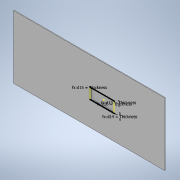
# Autodesk Inventor part: DecupajAgatare
Saved by Autodesk Inventor 2022 (Build 260153000, 153)
## iProperties
Created: 2022-04-14
Part Number: DecupajAgatare
Material: Generic
Document SubType Name: Sheet Metal
Designer: Janina
Density: 1 g/cm^3
Sheet Metal Rule: Default_mm
Appearance: Default
Author: Janina
Autodesk Inventor part; units mm, degrees
ref_plane "YZ Plane" through (0, 0, 0) normal (1, 0, 0) x (0, 1, 0)
ref_plane "XZ Plane" through (0, 0, 0) normal (0, 1, 0) x (-1, 0, 0)
ref_plane "XY Plane" through (0, 0, 0) normal (0, 0, 1) x (1, 0, 0)
sketch "Sketch1" plane through (0, 0, 0) normal (0, 0, 1) x (1, 0, 0)
  line L0 (-71.5423, 25.4266) -> (48.4577, 25.4266)
  line L1 (48.4577, 25.4266) -> (48.4577, -24.5734)
  line L2 (48.4577, -24.5734) -> (-71.5423, -24.5734)
  line L3 (-71.5423, -24.5734) -> (-71.5423, 25.4266)
  point P0 (0, 0)
  dimension "d0" = 50
  dimension "d1" = 120
  measures "d0" distance of L0.end L1.end
  measures "d1" distance of L0.start L0.end
extrude "Plate1" add sketch "Sketch1" along normal blind 0.5
sketch "Sketch2" plane through (0, 0, 0.5) normal (0, 0, 1) x (1, 0, 0)
  line L0 (-11.3208, 3.0189) -> (8.6792, 3.0189)
  line L1 (8.6792, 3.0189) -> (8.6792, -4.9811)
  line L2 (8.6792, -4.9811) -> (-11.3208, -4.9811)
  line L3 (-11.3208, -4.9811) -> (-11.3208, 3.0189)
  point P0 (0, 0)
  point P1 (-1.3208, -0.9811)
  dimension "LG_G" = 20
  dimension "LT_G" = 8
  dimension "d5" = 4
  dimension "d6" = 10
  constraints: 8 end point, 2 parallel, 1 horizontal, 1 perpendicular
  measures "LG_G" distance of L0.start L0.end
  measures "LT_G" distance of L0.end L1.end
  measures "d5" distance from line of L2 point (-1.321, -0.981)
  measures "d6" distance from line of L3 point (-1.321, -0.981)
extrude "Extrusion1" add sketch "Sketch2" against normal blind 1.5
sketch "Sketch3" plane through (0, 0, 0.5) normal (0, 0, 1) x (1, 0, 0)
  line L0 (-11.3208, 3.0189) -> (8.6792, 3.0189) projected
  line L1 (8.6792, 3.0189) -> (8.6792, -4.9811) projected
  line L2 (8.6792, -4.9811) -> (-11.3208, -4.9811) projected
  line L3 (-11.3208, -4.9811) -> (-11.3208, 3.0189) projected
  line L4 (-10.8208, 3.0189) -> (8.1792, 3.0189)
  line L5 (8.1792, 3.0189) -> (8.1792, -4.9811)
  line L6 (8.1792, -4.9811) -> (-10.8208, -4.9811)
  line L7 (-10.8208, -4.9811) -> (-10.8208, 3.0189)
  point P0 (0, 0)
  dimension "d9" = 0.5
  dimension "d10" = 0.5
  constraints: 8 end point, 2 collinear, 2 parallel, 1 horizontal, 1 perpendicular
  measures "d9" distance between parallel lines of L1 L5
  measures "d10" distance between parallel lines of L3 L7
extrude "Extrusion2" cut sketch "Sketch3" against normal blind 1 contours L0 L5 L2 L7
sketch "Sketch4" plane through (0, 0, 0.5) normal (0, 0, 1) x (1, 0, 0)
  line L0 (-10.8208, -4.9811) -> (-10.8208, 3.0189) projected
  line L1 (-10.8208, 3.0189) -> (8.1792, 3.0189) projected
  line L2 (8.1792, 3.0189) -> (8.1792, -4.9811) projected
  line L3 (8.1792, -4.9811) -> (-10.8208, -4.9811) projected
  line L4 (-11.3208, 3.5189) -> (8.6792, 3.5189)
  line L5 (8.6792, 3.5189) -> (8.6792, 3.0189)
  line L6 (8.6792, 3.0189) -> (-11.3208, 3.0189)
  line L7 (-11.3208, 3.0189) -> (-11.3208, 3.5189)
  line L8 (-11.3208, -4.9811) -> (8.6792, -4.9811)
  line L9 (8.6792, -4.9811) -> (8.6792, -5.4811)
  line L10 (8.6792, -5.4811) -> (-11.3208, -5.4811)
  line L11 (-11.3208, -5.4811) -> (-11.3208, -4.9811)
  point P0 (0, 0)
  dimension "d13" = 0.5
  dimension "d14" = 0.5
  dimension "d15" = 0.5
  dimension "d16" = 0.5
  constraints: 16 end point, 4 parallel, 2 collinear, 2 horizontal, 2 perpendicular, 2 point on line
  measures "d13" distance of L4.end L5.end
  measures "d14" distance of L8.end L9.end
  measures "d15" distance between parallel lines of L7 L0
  measures "d16" distance between parallel lines of L2 L5
equation "\"d5\" = 0.5 * LT_G"
equation "\"d6\" = 0.5 * LG_G"
equation "\"d7\" = 3 * Thickness"
equation "\"d9\" = Thickness"
equation "\"d10\" = Thickness"
equation "\"d11\" = 2 * Thickness"
equation "\"d13\" = Thickness"
equation "\"d14\" = Thickness"
equation "\"d15\" = Thickness"
equation "\"d16\" = Thickness"
equation "\"d2\" = Thickness"
equation "\"BendRadius\" = Thickness"
equation "\"BendReliefWidth\" = Thickness"
equation "\"BendReliefDepth\" = 0.5 * Thickness"
equation "\"CornerReliefSize\" = 4 * Thickness"
equation "\"MinimumRemnant\" = 2 * Thickness"
equation "\"TransitionRadius\" = BendRadius"
equation "\"JacobiRadiusSize\" = BendRadius"
equation "\"GapSize\" = Thickness"
equation "\"Thickness\" = 0.5"
body "Solid1"
